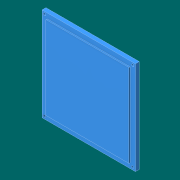
# Autodesk Inventor part: back
Saved by Autodesk Inventor 2016 (Build 200138000, 138)
## iProperties
Created: 2015-10-13
Part Number: back
Material: PC/ABS Plastic
Document SubType Name: Modeling
Designer: Sawaiz
Density: 0.357273 g/cm^3
Appearance: Cyan
Author: Sawaiz
Autodesk Inventor part; units mm, degrees
ref_plane "YZ Plane" through (0, 0, 0) normal (1, 0, 0) x (0, 1, 0)
ref_plane "XZ Plane" through (0, 0, 0) normal (0, 1, 0) x (-1, 0, 0)
ref_plane "XY Plane" through (0, 0, 0) normal (0, 0, 1) x (1, 0, 0)
sketch "Sketch1" plane through (0, 0, 0) normal (1, 0, 0) x (0, 1, 0)
  line L0 (-57.15, -57.15) -> (57.15, -57.15)
  line L1 (57.15, -57.15) -> (57.15, 57.15)
  line L2 (57.15, 57.15) -> (-57.15, 57.15)
  line L3 (-57.15, 57.15) -> (-57.15, -57.15)
  line L4 (-57.15, -57.15) -> (57.15, 57.15) construction
  line L5 (57.15, -57.15) -> (-57.15, 57.15) construction
  point P0 (0, 0)
  dimension "d0" = 114.3
  dimension "d1" = 114.3
  constraints: 12 end point, 2 midpoint, 2 parallel, 1 horizontal, 1 perpendicular
  measures "d0" distance of L2.end L1.end
  measures "d1" distance of L1.end L0.end
extrude "Extrusion1" add sketch "Sketch1" along normal blind 6.35
sketch "Sketch4" plane through (0, 0, 0) normal (-1, 0, 0) x (0, 0, 1)
  line L0 (-57.15, -57.15) -> (-57.15, 57.15) projected
  line L1 (57.15, -57.15) -> (-57.15, -57.15) projected
  line L2 (57.15, 57.15) -> (57.15, -57.15) projected
  line L3 (-57.15, 57.15) -> (57.15, 57.15) projected
  line L4 (57.15, 57.15) -> (57.15, -57.15) projected
  line L5 (-57.15, 57.15) -> (57.15, 57.15) projected
  line L6 (-53.975, 53.975) -> (53.975, 53.975)
  line L7 (53.975, 53.975) -> (53.975, -53.975)
  line L8 (53.975, -53.975) -> (-53.975, -53.975)
  line L9 (-53.975, -53.975) -> (-53.975, 53.975)
  line L10 (-53.975, 53.975) -> (53.975, -53.975) construction
  line L11 (53.975, 53.975) -> (-53.975, -53.975) construction
  point P0 (0, 0)
  dimension "d83" = 3.175
  dimension "d84" = 3.175
  constraints: 12 end point, 4 coincident, 2 midpoint, 2 parallel, 1 horizontal, 1 perpendicular
  measures "d83" distance between parallel lines of L3 L6
  measures "d84" distance between parallel lines of L2 L7
hole "Hole1" at (0, 53.975, 53.975) at (0, 53.975, -53.975) at (0, -53.975, -53.975) at (0, -53.975, 53.975) direction (1, 0, 0) diameter 2.946 end through all countersink diameter 5.715 countersink angle 82 clearance for "Flat Head Machine Screw (82)" size "#4" standard "Ansi Unified Screw Threads"
sketch "Sketch10" plane through (6.35, 0, 0) normal (1, 0, 0) x (0, 0, -1)
  line L0 (50.8, -50.8) -> (-50.8, -50.8)
  line L1 (-50.8, -50.8) -> (-50.8, 50.8)
  line L2 (-50.8, 50.8) -> (50.8, 50.8)
  line L3 (50.8, 50.8) -> (50.8, -50.8)
  line L4 (50.8, -50.8) -> (-50.8, 50.8) construction
  line L5 (-50.8, -50.8) -> (50.8, 50.8) construction
  circle A0 centre (53.975, -53.975) radius 1.473 projected
  circle A1 centre (-53.975, 53.975) radius 1.473 projected
  circle A2 centre (53.975, 53.975) radius 1.473 projected
  circle A3 centre (-53.975, -53.975) radius 1.473 projected
  line L6 (57.15, -57.15) -> (57.15, 57.15) projected
  line L7 (57.15, 57.15) -> (-57.15, 57.15) projected
  line L8 (-57.15, 57.15) -> (-57.15, -57.15) projected
  line L9 (-57.15, -57.15) -> (57.15, -57.15) projected
  point P0 (0, 0)
  dimension "d125" = 101.6
  dimension "d126" = 101.6
  constraints: 12 end point, 2 midpoint, 2 parallel, 1 horizontal, 1 perpendicular
  measures "d125" distance of L1.end L2.end
  measures "d126" distance of L0.end L1.end
extrude "Extrusion5" cut sketch "Sketch10" against normal blind 1.5875
equation "\"d0\" = height + 2 * acrylicThickness"
equation "\"d1\" = height + 2 * acrylicThickness"
equation "\"acrylicThickness\" = 6.35"
equation "\"height\" = 101.6"
equation "\"width\" = 101.6"
equation "\"depth\" = 152.4"
equation "\"mirrorAngle\" = 5deg"
equation "\"detectorWidth\" = 52"
equation "\"detectorHeight\" = 52"
equation "\"mirrorThickness\" = 3.175"
equation "\"fresnelThickness\" = 0.1"
equation "\"ior\" = 1.49"
equation "\"focalLength\" = 76.2"
equation "\"fresnelAngle\" = 90deg"
equation "\"centerThickness\" = 1.524"
equation "\"fresnelEffectiveDiameter\" = 76.2"
equation "\"mirrorSuppourtWidth\" = 38.1"
equation "\"backGrooveBit\" = 4.8006"
equation "\"sensorHolderHeight\" = 88.9"
equation "\"sensorHolderWidth\" = 88.9"
equation "\"sensorHolderSensorWidth\" = 53.975"
equation "\"sensorHolderSesnorHeight\" = 53.975"
equation "\"sensorHolderSensorHeight\" = 53.975"
equation "\"sensorHolderORingGroove\" = 3.175"
equation "\"sensorHolderORing\" = 3.175"
equation "\"sensorHolderFlushORingID\" = 304.8"
equation "\"sensorHolderFlushORing\" = 3.175"
equation "\"sensorHolderORingID\" = 203.2"
equation "\"oRingWidth\" = 3.175"
equation "\"frontBackORingID\" = 419.1"
equation "\"topBottomHorizontalMirrorGroove\" = 12.7"
equation "\"backMirrorGroove\" = 6.35"
equation "\"mirrorGroove\" = 19.05"
equation "\"fresnelChamfer\" = 6.35"
equation "\"mirrorGrooveFillet\" = 6.35"
equation "\"mirrorGrooveDrill\" = 6.35"
equation "\"mirrorGrooveMill\" = 3.175"
equation "\"fresnelMirrorChamfer\" = 6.35"
equation "\"detectorOpeningWidth\" = 76.2"
equation "\"detectorOpeningHeight\" = 76.2"
body "Solid1"
